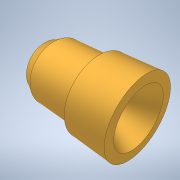
# Autodesk Inventor part: Сопло фильеры
Saved by Autodesk Inventor 2021.1 (Build 251245010, 245A)
## iProperties
Created: 2026-05-28
Part Number: Сопло фильеры
Material: Типовые
Document SubType Name: Modeling
Designer: Андрей Тарасов
Density: 1 g/cm^3
Appearance: По умолчанию
Author: Андрей Тарасов
Autodesk Inventor part; units mm, degrees
ref_plane "YZ Plane" through (0, 0, 0) normal (1, 0, 0) x (0, 1, 0)
ref_plane "XZ Plane" through (0, 0, 0) normal (0, 1, 0) x (-1, 0, 0)
ref_plane "XY Plane" through (0, 0, 0) normal (0, 0, 1) x (1, 0, 0)
sketch "Эскиз1" plane through (0, 0, 0) normal (0, 0, 1) x (1, 0, 0)
  line L0 (1, 0.1) -> (0, 1.1)
  line L1 (0, 1.1) -> (0, 3.35)
  line L2 (0, 3.35) -> (1.7, 4.1)
  line L3 (1.7, 4.1) -> (8, 4.1)
  line L4 (8, 4.1) -> (8, 4.85)
  line L5 (8, 4.85) -> (13, 4.85)
  line L6 (13, 4.85) -> (13, 3.65)
  line L7 (13, 3.65) -> (6, 0.1)
  line L8 (6, 0.1) -> (1, 0.1)
  line L9 (-2.6, 0) -> (15.6, 0) construction
  line L10 (0, -0.97) -> (0, 5.82) construction
  point P0 (0, 0)
  point P1 (0, -0.97)
  dimension "d1" = 0.1
  dimension "d2" = 4.1
  dimension "d3" = 1.7
  dimension "d5" = 3.35
  dimension "d6" = 1
  dimension "d7" = 135
  dimension "d8" = 5
  dimension "d9" = 13
  dimension "d10" = 4.85
  dimension "d11" = 5
  dimension "d12" = 1.2
  constraints: 18 end point, 2 perpendicular, 2 vertical, 1 horizontal, 1 other
  measures "d1" distance between parallel lines of L8 L9
  measures "d2" distance between parallel lines of L3 L9
  measures "d3" distance from line of L2.end L1
  measures "d5" distance from line of L9 L1.end
  measures "d6" distance from line of L1 L0.start
  measures "d7" angle of L1 L0
  measures "d8" distance of L4.end L5.end
  measures "d9" distance between parallel lines of L6 L1
  measures "d10" distance between parallel lines of L9 L5
  measures "d11" distance of L7.end L0.start
  measures "d12" distance of L5.end L6.end
revolve "Вращение1" add sketch "Эскиз1" angle 360 about axis through (-10, 0, 0) along (1, 0, 0)
